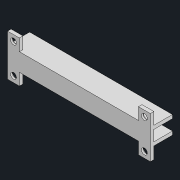
# Autodesk Inventor part: RackSlider
Saved by Autodesk Inventor 2022.2 (Build 262287010, 287A)
## iProperties
Created: 2022-06-04
Part Number: RackSlider
Material: Generic
Document SubType Name: Modeling
Designer: frede
Density: 1 g/cm^3
Appearance: Default
ScrewPlateSize: 10.000 mm
ScrewPlateHeight: 3.000 mm
ScrewHoleDia: 5.000 mm
ScrewHoleFillet: 1.500 mm
RackOffset: 0.500 mm
Author: frede
Autodesk Inventor part; units mm, degrees
ref_plane "YZ Plane" through (0, 0, 0) normal (1, 0, 0) x (0, 1, 0)
ref_plane "XZ Plane" through (0, 0, 0) normal (0, 1, 0) x (-1, 0, 0)
ref_plane "XY Plane" through (0, 0, 0) normal (0, 0, 1) x (1, 0, 0)
sketch "Sketch1" plane through (0, 0, 0) normal (1, 0, 0) x (0, 1, 0)
  line L0 (4.5, -15.6) -> (4.5, 0)
  line L1 (4.5, 0) -> (-4.5, 0)
  line L2 (-4.5, 0) -> (-4.5, -15.6)
  line L3 (7.5, -15.6) -> (7.5, 3)
  line L4 (7.5, 3) -> (-7.5, 3)
  line L5 (-7.5, 3) -> (-7.5, -15.6)
  line L6 (-7.5, -15.6) -> (-4.5, -15.6)
  line L7 (4.5, -15.6) -> (7.5, -15.6)
  point P0 (0, 0)
  point P1 (0, 0)
  dimension "SliderWallWidth" = 3
  dimension "d18" = 9
  dimension "d19" = 15.6
  constraints: 16 end point, 3 horizontal, 3 horizontal alignment, 2 parallel, 1 coincident, 1 midpoint, 1 vertical, 2 other
  measures "SliderWallWidth" distance between parallel lines of L2 L5
  measures "d18" distance between parallel lines of L2 L0
  measures "d19" distance of L0.start L0.end
extrude "Extrusion1" add sketch "Sketch1" along normal mid plane 120
sketch "Sketch2" plane through (-60, -7.5, -15.6) normal (0, -1, 0) x (1, 0, 0)
  line L0 (120, 18.6) -> (110, 18.6)
  line L1 (110, 18.6) -> (110, 15.6)
  line L2 (110, 15.6) -> (120, 15.6)
  line L3 (120, 15.6) -> (120, 18.6)
  dimension "ScrewPlateSize" = 10
  dimension "ScrewPlateHeight" = 3
  constraints: 8 end point, 2 parallel, 1 horizontal, 1 perpendicular
  measures "ScrewPlateSize" distance of L2.end L1.end
  measures "ScrewPlateHeight" distance of L1.end L0.end
extrude "Extrusion2" add sketch "Sketch2" along normal blind 10
sketch "Sketch5" plane through (60, -7.5, 0) normal (0, 0, -1) x (-1, 0, 0)
  line L0 (10, -10) -> (0, -10) construction
  line L1 (10, 0) -> (10, -10) construction
  circle A0 centre (5, -5) radius 2.5
  point P0 (60, 7.5)
  point P1 (10, -5)
  point P2 (5, -10)
  dimension "ScrewHoleDia" = 5
  constraints: 2 midpoint, 1 centre point, 1 horizontal alignment, 1 vertical alignment
  measures "ScrewHoleDia" diameter of A0
extrude "Extrusion4" cut sketch "Sketch5" against normal through all
chamfer "Chamfer2" distance 1.5 angle 45 1 edges at (57.5, -12.5, 0)
mirror "Mirror2" about plane through (0, 0, 0) normal (0, 1, 0) of "Extrusion4", "Chamfer2", "Extrusion2"
mirror "Mirror3" about plane through (0, 0, 0) normal (1, 0, 0) of "Extrusion4", "Chamfer2", "Extrusion2", "Mirror2"
equation "\"d18\" = RackWidth + 2 * RackOffset"
equation "\"d19\" = RackHeight"
equation "\"d3\" = RackLength"
equation "\"d9\" = ScrewPlateSize"
equation "\"RackOffset\" = 0.5"
equation "\"RackWidth\" = 8"
equation "\"RackHeight\" = 15.6"
equation "\"RackLength\" = 120"
body "Solid1"
